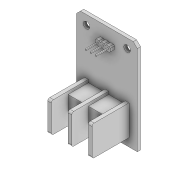
# Autodesk Inventor part: current sensor
Saved by Autodesk Inventor 2020.3 (Build 243373000, 373)
## iProperties
Created: 2020-11-25
Part Number: current sensor
Material: Generic
Document SubType Name: Modeling
Designer: Svend
Density: 1 g/cm^3
Appearance: Default
Author: Svend
Autodesk Inventor part; units mm, degrees
ref_plane "YZ Plane" through (0, 0, 0) normal (1, 0, 0) x (0, 1, 0)
ref_plane "XZ Plane" through (0, 0, 0) normal (0, 1, 0) x (-1, 0, 0)
ref_plane "XY Plane" through (0, 0, 0) normal (0, 0, 1) x (1, 0, 0)
sketch "Sketch1" plane through (0, 0, 0) normal (0, 0, 1) x (1, 0, 0)
  line L0 (-13, 23) -> (13, 23)
  line L1 (15, 21) -> (15, -23)
  line L2 (15, -23) -> (-15, -23)
  line L3 (-15, -23) -> (-15, 21)
  line L4 (-15, 23) -> (15, -23) construction
  line L5 (15, 23) -> (-15, -23) construction
  line L6 (-13, 23) -> (-15, 21)
  line L7 (13, 23) -> (15, 21)
  circle A0 centre (-10, 18.5) radius 1.6
  circle A1 centre (10, 18.5) radius 1.6
  line L8 (10, 18.5) -> (-10, 18.5) construction
  point P0 (0, 0)
  point P1 (0, 18.5)
  point P2 (0, 0)
  dimension "d0" = 30
  dimension "d1" = 46
  dimension "d2" = 2
  dimension "d3" = 2
  dimension "d4" = 2
  dimension "d5" = 2
  dimension "d6" = 3.2
  dimension "d7" = 20
  dimension "d8" = 4.5
  constraints: 18 end point, 4 midpoint, 4 point on line, 2 centre point, 2 horizontal, 2 parallel, 1 equal radius, 1 horizontal alignment, 1 perpendicular, 1 vertical alignment
  measures "d0" distance of L1.end L2.end
  measures "d1" distance of L5.start L1.end
  measures "d2" distance of L0.start L4.start
  measures "d3" distance of L3.end L4.start
  measures "d4" distance of L0.end L5.start
  measures "d5" distance of L1.start L5.start
  measures "d6" diameter of A1
  measures "d7" distance of L8.start L8.end
  measures "d8" distance from line of L0 L8.start
extrude "Extrusion1" add sketch "Sketch1" along normal blind 1.6
sketch "Sketch2" plane through (0, 0, 1.6) normal (0, 0, 1) x (1, 0, 0)
  line L0 (10.9, -19) -> (9.1, -19)
  line L1 (9.1, -19) -> (9.1, -4.2)
  line L2 (9.1, -4.2) -> (10.9, -4.2)
  line L3 (10.9, -4.2) -> (10.9, -19)
  line L4 (0.9, -19) -> (-0.9, -19)
  line L5 (-0.9, -19) -> (-0.9, -4.2)
  line L6 (-0.9, -4.2) -> (0.9, -4.2)
  line L7 (0.9, -4.2) -> (0.9, -19)
  line L8 (-9.1, -19) -> (-10.9, -19)
  line L9 (-10.9, -19) -> (-10.9, -4.2)
  line L10 (-10.9, -4.2) -> (-9.1, -4.2)
  line L11 (-9.1, -4.2) -> (-9.1, -19)
  line L12 (-15, 21) -> (-15, -23) projected
  line L13 (-15, -23) -> (15, -23) projected
  line L14 (15, -23) -> (15, 21) projected
  line L15 (15, 21) -> (13, 23) projected
  line L16 (13, 23) -> (-13, 23) projected
  line L17 (-13, 23) -> (-15, 21) projected
  circle A0 centre (10, 18.5) radius 1.6 projected
  circle A1 centre (-10, 18.5) radius 1.6 projected
  line L18 (-0.9, -4.2) -> (0.9, -19) construction
  line L19 (0.9, -4.2) -> (-0.9, -19) construction
  line L20 (10.9, -4.2) -> (9.1, -19) construction
  line L21 (9.1, -4.2) -> (10.9, -19) construction
  line L22 (-10.9, -4.2) -> (-9.1, -19) construction
  line L23 (-9.1, -4.2) -> (-10.9, -19) construction
  point P0 (0, 0)
  point P1 (0, -11.6)
  dimension "d11" = 1.8
  dimension "d12" = 14.8
  dimension "d13" = 4
  dimension "d14" = 8.2
  dimension "d15" = 8.2
  constraints: 36 end point, 10 parallel, 4 point on line, 3 horizontal, 3 perpendicular, 2 collinear, 1 midpoint, 1 vertical alignment
  measures "d11" distance of L5.end L6.end
  measures "d12" distance of L6.end L4.start
  measures "d13" distance between parallel lines of L13 L0
  measures "d14" distance between parallel lines of L1 L7
  measures "d15" distance between parallel lines of L11 L5
extrude "Extrusion2" add sketch "Sketch2" along normal blind 18.2 contours L0 L1 L2 L3 | L4 L5 L6 L7 | L8 L9 L10 L11
fillet "Fillet1" radius 1 6 edges at (-10, -19, 19.8) (-10, -4.2, 19.8) (0, -4.2, 19.8) (0, -19, 19.8) (10, -19, 19.8) (10, -4.2, 19.8)
sketch "Sketch3" plane through (9.1, -19, 1.6) normal (-1, 0, 0) x (0, 0, 1)
  arc A0 (18.2, 13.8) -> (17.2, 14.8) centre (17.2, 13.8) ccw projected
  line L0 (0, 14.8) -> (17.2, 14.8) projected
  line L1 (0, 0) -> (0, 14.8) projected
  line L2 (0, 0) -> (17.2, 0) projected
  arc A1 (17.2, 0) -> (18.2, 1) centre (17.2, 1) ccw projected
  line L3 (18.2, 13.8) -> (18.2, 1) projected
  line L4 (0, 0) -> (0, 14.8) projected
  line L5 (10, 13.4) -> (0, 13.4)
  line L6 (0, 13.4) -> (0, 1.4)
  line L7 (0, 1.4) -> (10, 1.4)
  line L8 (10, 1.4) -> (10, 13.4)
  line L9 (10, 13.4) -> (0, 1.4) construction
  line L10 (0, 13.4) -> (10, 1.4) construction
  point P0 (-1.6, 19)
  point P1 (5, 7.4)
  point P2 (5, 7.4)
  point P3 (18.2, 7.4)
  point P4 (0, 13.4)
  point P5 (0, 1.4)
  dimension "d19" = 10
  dimension "d20" = 12
  constraints: 12 end point, 4 midpoint, 2 parallel, 1 horizontal, 1 horizontal alignment, 1 perpendicular, 1 point on line
  measures "d19" distance of L6.end L7.end
  measures "d20" distance of L7.end L5.start
extrude "Extrusion3" add sketch "Sketch3" along normal up to surface (18.2 mm away) contours L5 L8 L7 L1
sketch "Sketch4" plane through (0, 0, 1.6) normal (0, 0, 1) x (1, 0, 0)
  circle A0 centre (-10, 18.5) radius 1.6 projected
  circle A1 centre (10, 18.5) radius 1.6 projected
  line L0 (-15, 21) -> (-15, -23) projected
  line L1 (-15, -23) -> (15, -23) projected
  line L2 (15, -23) -> (15, 21) projected
  line L3 (15, 21) -> (13, 23) projected
  line L4 (13, 23) -> (-13, 23) projected
  line L5 (-13, 23) -> (-15, 21) projected
  line L6 (-0.9, -17.6) -> (-9.1, -17.6) projected
  line L7 (-9.1, -17.6) -> (-9.1, -19) projected
  line L8 (-9.1, -19) -> (-10.9, -19) projected
  line L9 (-10.9, -19) -> (-10.9, -4.2) projected
  line L10 (-10.9, -4.2) -> (-9.1, -4.2) projected
  line L11 (-9.1, -4.2) -> (-9.1, -5.6) projected
  line L12 (-9.1, -5.6) -> (-0.9, -5.6) projected
  line L13 (-0.9, -5.6) -> (-0.9, -4.2) projected
  line L14 (-0.9, -4.2) -> (0.9, -4.2) projected
  line L15 (0.9, -4.2) -> (0.9, -5.6) projected
  line L16 (0.9, -5.6) -> (9.1, -5.6) projected
  line L17 (9.1, -5.6) -> (9.1, -4.2) projected
  line L18 (9.1, -4.2) -> (10.9, -4.2) projected
  line L19 (10.9, -4.2) -> (10.9, -19) projected
  line L20 (10.9, -19) -> (9.1, -19) projected
  line L21 (9.1, -19) -> (9.1, -17.6) projected
  line L22 (9.1, -17.6) -> (0.9, -17.6) projected
  line L23 (0.9, -17.6) -> (0.9, -19) projected
  line L24 (0.9, -19) -> (-0.9, -19) projected
  line L25 (-0.9, -19) -> (-0.9, -17.6) projected
  line L26 (0.75, 17) -> (-0.75, 17)
  line L27 (-1.25, 16.5) -> (-1.25, 15)
  line L28 (-0.75, 14.5) -> (0.75, 14.5)
  line L29 (1.25, 15) -> (1.25, 16.5)
  line L30 (1.25, 16.5) -> (0.75, 17)
  line L31 (1.25, 15) -> (0.75, 14.5)
  line L32 (-0.75, 14.5) -> (-1.25, 15)
  line L33 (-1.25, 16.5) -> (-0.75, 17)
  line L34 (-3.75, 16.5) -> (-3.25, 17)
  line L35 (-3.75, 16.5) -> (-3.75, 15)
  line L36 (-3.25, 14.5) -> (-3.75, 15)
  line L37 (-1.75, 17) -> (-3.25, 17)
  line L38 (-3.25, 14.5) -> (-1.75, 14.5)
  line L39 (-1.25, 15) -> (-1.75, 14.5)
  line L40 (-1.25, 15) -> (-1.25, 16.5)
  line L41 (-1.25, 16.5) -> (-1.75, 17)
  line L42 (1.25, 16.5) -> (1.75, 17)
  line L43 (1.25, 16.5) -> (1.25, 15)
  line L44 (1.75, 14.5) -> (1.25, 15)
  line L45 (3.25, 17) -> (1.75, 17)
  line L46 (1.75, 14.5) -> (3.25, 14.5)
  line L47 (3.75, 15) -> (3.25, 14.5)
  line L48 (3.75, 15) -> (3.75, 16.5)
  line L49 (3.75, 16.5) -> (3.25, 17)
  line L50 (-1.25, 16.5) -> (-0.75, 17)
  line L51 (-1.25, 16.5) -> (-1.25, 15)
  line L52 (-0.75, 14.5) -> (-1.25, 15)
  line L53 (0.75, 17) -> (-0.75, 17)
  line L54 (-0.75, 14.5) -> (0.75, 14.5)
  line L55 (1.25, 15) -> (0.75, 14.5)
  line L56 (1.25, 15) -> (1.25, 16.5)
  line L57 (1.25, 16.5) -> (0.75, 17)
  point P0 (0, 0)
  point P1 (1.25, 17)
  point P2 (-1.25, 14.5)
  point P3 (-1.25, 17)
  point P4 (1.25, 14.5)
  point P5 (0, 17)
  point P6 (0, 23)
  point P7 (-3.75, 17)
  point P8 (-3.75, 14.5)
  point P9 (-2.5, 17)
  point P10 (-1.25, 17)
  point P11 (-1.25, 14.5)
  point P12 (1.25, 17)
  point P13 (1.25, 14.5)
  point P14 (2.5, 17)
  point P15 (3.75, 17)
  point P16 (3.75, 14.5)
  point P17 (-1.25, 17)
  point P18 (-1.25, 14.5)
  point P19 (0, 17)
  point P20 (1.25, 17)
  point P21 (1.25, 14.5)
  dimension "d23" = 2.5
  dimension "d24" = 2.5
  dimension "d25" = 0.5
  dimension "d26" = 0.5
  dimension "d27" = 0.5
  dimension "d28" = 0.5
  dimension "d29" = 0.5
  dimension "d30" = 0.5
  dimension "d31" = 0.5
  dimension "d32" = 0.5
  dimension "d33" = 6
  dimension "d36" = 2.5
  dimension "d39" = 2.5
  constraints: 64 end point, 32 point on line, 3 horizontal, 2 midpoint, 2 parallel, 1 perpendicular, 1 vertical alignment, 63 other
  measures "d23" distance of point (1.25, 14.5) point (-1.25, 14.5)
  measures "d24" distance of point (-1.25, 14.5) point (-1.25, 17)
  measures "d25" distance of L29.end point (1.25, 17)
  measures "d26" distance of L26.start point (1.25, 17)
  measures "d27" distance of L29.start point (1.25, 14.5)
  measures "d28" distance of L28.end point (1.25, 14.5)
  measures "d29" distance of L28.start point (-1.25, 14.5)
  measures "d30" distance of L27.end point (-1.25, 14.5)
  measures "d31" distance of L27.start point (-1.25, 17)
  measures "d32" distance of L26.end point (-1.25, 17)
  measures "d33" distance between parallel lines of L4 L26
  measures "d36" distance of point (-1.25, 17) point (-3.75, 17)
  measures "d39" distance of point (-1.25, 17) point (1.25, 17)
extrude "Extrusion4" add sketch "Sketch4" along normal blind 2 contours L30 L29 L31 L28 L32 L27 L33 L26 | L42 L45 L49 L48 L47 L46 L44 L29 | L27 L39 L38 L36 L35 L34 L37 L41
sketch "Sketch5" plane through (0, 0, 3.6) normal (0, 0, 1) x (1, 0, 0)
  line L0 (1.25, 16.5) -> (0.75, 17) projected
  line L1 (0.75, 17) -> (-0.75, 17) projected
  line L2 (-0.75, 17) -> (-1.25, 16.5) projected
  line L3 (-1.25, 16.5) -> (-1.75, 17) projected
  line L4 (-1.75, 17) -> (-3.25, 17) projected
  line L5 (-3.25, 17) -> (-3.75, 16.5) projected
  line L6 (-3.75, 16.5) -> (-3.75, 15) projected
  line L7 (-3.75, 15) -> (-3.25, 14.5) projected
  line L8 (-3.25, 14.5) -> (-1.75, 14.5) projected
  line L9 (-1.75, 14.5) -> (-1.25, 15) projected
  line L10 (-1.25, 15) -> (-0.75, 14.5) projected
  line L11 (-0.75, 14.5) -> (0.75, 14.5) projected
  line L12 (0.75, 14.5) -> (1.25, 15) projected
  line L13 (1.25, 15) -> (1.75, 14.5) projected
  line L14 (1.75, 14.5) -> (3.25, 14.5) projected
  line L15 (3.25, 14.5) -> (3.75, 15) projected
  line L16 (3.75, 15) -> (3.75, 16.5) projected
  line L17 (3.75, 16.5) -> (3.25, 17) projected
  line L18 (3.25, 17) -> (1.75, 17) projected
  line L19 (1.75, 17) -> (1.25, 16.5) projected
  line L20 (-3.75, 16.5) -> (-3.75, 15) projected
  line L21 (2.75, 15.5) -> (2.25, 15.5)
  line L22 (2.25, 15.5) -> (2.25, 16)
  line L23 (2.25, 16) -> (2.75, 16)
  line L24 (2.75, 16) -> (2.75, 15.5)
  line L25 (2.75, 15.5) -> (2.25, 16) construction
  line L26 (2.25, 15.5) -> (2.75, 16) construction
  line L27 (0.25, 15.5) -> (-0.25, 15.5)
  line L28 (-0.25, 15.5) -> (-0.25, 16)
  line L29 (-0.25, 16) -> (0.25, 16)
  line L30 (0.25, 16) -> (0.25, 15.5)
  line L31 (0.25, 15.5) -> (-0.25, 16) construction
  line L32 (-0.25, 15.5) -> (0.25, 16) construction
  line L33 (-2.25, 15.5) -> (-2.75, 15.5)
  line L34 (-2.75, 15.5) -> (-2.75, 16)
  line L35 (-2.75, 16) -> (-2.25, 16)
  line L36 (-2.25, 16) -> (-2.25, 15.5)
  line L37 (-2.25, 15.5) -> (-2.75, 16) construction
  line L38 (-2.75, 15.5) -> (-2.25, 16) construction
  point P0 (0, 0)
  point P1 (2.5, 15.75)
  point P2 (0, 15.75)
  point P3 (-2.5, 15.75)
  point P4 (2.5, 14.5)
  point P5 (0, 14.5)
  point P6 (-2.5, 14.5)
  point P7 (-3.75, 15.75)
  point P8 (-3.75, 15.75)
  point P9 (3.75, 15.75)
  dimension "d44" = 0.5
  dimension "d45" = 0.5
  dimension "d46" = 0.5
  dimension "d47" = 0.5
  dimension "d48" = 0.5
  dimension "d49" = 0.5
  constraints: 36 end point, 12 midpoint, 6 parallel, 3 horizontal, 3 horizontal alignment, 3 perpendicular, 3 vertical alignment
  measures "d44" distance of L22.end L23.end
  measures "d45" distance of L21.end L22.end
  measures "d46" distance of L28.end L29.end
  measures "d47" distance of L27.end L28.end
  measures "d48" distance of L34.end L35.end
  measures "d49" distance of L33.end L34.end
extrude "Extrusion5" add sketch "Sketch5" along normal blind 6 contours L21 L22 L23 L24 | L27 L28 L29 L30 | L33 L34 L35 L36
equation "\"d3\" = d2"
equation "\"d4\" = d2"
equation "\"d5\" = d4"
equation "\"d15\" = d14"
equation "\"d26\" = d25"
equation "\"d27\" = d25"
equation "\"d28\" = d27"
equation "\"d29\" = d25"
equation "\"d30\" = d29"
equation "\"d31\" = d25"
equation "\"d32\" = d31"
body "Solid1"
